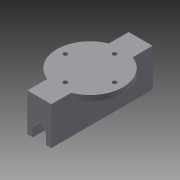
# Autodesk Inventor part: CarFrontAxel
Saved by Autodesk Inventor 2015 (Build 190159000, 159)
## iProperties
Created: 2016-04-06
Part Number: CarFrontAxel
Material: Generic
Document SubType Name: Modeling
Designer: Lee
Density: 1 g/cm^3
Appearance: Default
Author: Lee
Autodesk Inventor part; units mm, degrees
ref_plane "YZ Plane" through (0, 0, 0) normal (1, 0, 0) x (0, 1, 0)
ref_plane "XZ Plane" through (0, 0, 0) normal (0, 1, 0) x (-1, 0, 0)
ref_plane "XY Plane" through (0, 0, 0) normal (0, 0, 1) x (1, 0, 0)
sketch "Sketch1" plane through (0, 0, 0) normal (0, 0, 1) x (1, 0, 0)
  line L0 (0, 0) -> (7.2, 0)
  line L1 (7.2, 0) -> (7.2, 30.48)
  line L2 (7.2, 30.48) -> (0, 30.48)
  line L3 (0, 30.48) -> (0, 0)
  line L4 (5.6, 28.88) -> (5.6, 1.6)
  line L5 (5.6, 1.6) -> (1.6, 1.6)
  line L6 (1.6, 1.6) -> (1.6, 28.88)
  line L7 (1.6, 28.88) -> (5.6, 28.88)
  dimension "d0" = 30.48
  dimension "d1" = 7.2
  dimension "d2" = 1.6
  constraints: 16 end point, 4 parallel, 2 perpendicular, 1 horizontal, 3 other
  measures "d0" distance of L0.end L1.end
  measures "d1" distance of L0.start L0.end
  measures "d2" distance between parallel lines of L1 L4
extrude "Extrusion1" add sketch "Sketch1" along normal blind 11.4
sketch "Sketch2" plane through (0, 0, 0) normal (0, -1, 0) x (1, 0, 0)
  line L0 (5.6, 0) -> (5.6, 11.4) projected
  line L1 (1.6, 0) -> (1.6, 11.4) projected
  line L2 (0, 0) -> (7.2, 0) projected
  line L3 (1.6, 0) -> (1.6, 2.4)
  line L4 (1.6, 0) -> (1.6, 11.4) projected
  line L5 (5.6, 0) -> (5.6, 2.4)
  line L6 (5.6, 0) -> (5.6, 11.4) projected
  line L7 (1.6, 0) -> (5.6, 0)
  arc A0 (5.6, 2.4) -> (1.6, 2.4) centre (3.6, 2.4) ccw
  dimension "d5" = 2.4
  dimension "d6" = 2.4
  constraints: 6 end point, 2 point on circle, 2 point on line, 1 centre point, 1 tangent
  measures "d5" distance of L1.start L3.end
  measures "d6" distance of L0.start L5.end
extrude "Extrusion2" cut sketch "Sketch2" against normal up to surface (30.48 mm away)
sketch "Sketch3" plane through (0, 0, 0) normal (-1, 0, 0) x (0, 0, 1)
  line L0 (0, 30.48) -> (0, 0) projected
  line L1 (0, 0) -> (11.4, 0) projected
  line L2 (11.4, 30.48) -> (11.4, 0) projected
  line L3 (0, 30.48) -> (11.4, 30.48) projected
  line L4 (0, 0) -> (11.4, 0) projected
  line L5 (11.4, 30.48) -> (9.8, 30.48)
  line L6 (9.8, 30.48) -> (9.8, 0)
  line L7 (9.8, 0) -> (11.4, 0)
  line L8 (11.4, 0) -> (11.4, 30.48)
  dimension "d9" = 1.6
  constraints: 8 end point, 2 parallel, 1 horizontal, 1 perpendicular, 1 point on line
  measures "d9" distance of L7.end L6.end
extrude "Extrusion3" add sketch "Sketch3" against normal up to next contours L3 L2 L1 L6
sketch "Sketch4" plane through (0, 0, 11.4) normal (0, 0, 1) x (1, 0, 0)
  line L0 (0, 0) -> (7.2, 0) projected
  line L1 (7.2, 0) -> (7.2, 30.48) projected
  line L2 (7.2, 30.48) -> (0, 30.48) projected
  line L3 (0, 30.48) -> (0, 0) projected
  line L4 (5.6, 0) -> (1.6, 0) projected
  line L5 (3.6, 0) -> (3.6, 30.48)
  line L6 (1.6, 30.48) -> (5.6, 30.48) projected
  line L7 (7.2, 0) -> (0, 30.48)
  line L8 (7.2, 30.48) -> (0, 0) construction
  circle A0 centre (3.6, 7.84) radius 0.65
  circle A1 centre (3.6, 22.64) radius 0.65
  point P0 (3.6, 15.24)
  dimension "d12" = 7.4
  dimension "d13" = 7.4
  dimension "d14" = 1.3
  dimension "d15" = 1.3
  constraints: 6 end point, 3 midpoint, 2 centre point, 2 point on line
  measures "d12" distance of point (3.6, 15.24) A0.centre
  measures "d13" distance of point (3.6, 15.24) A1.centre
  measures "d14" diameter of A0
  measures "d15" diameter of A1
extrude "Extrusion4" cut sketch "Sketch4" against normal up to next contours A0 L5 | L5 A0 | A1 L5 | L5 A1
sketch "Sketch5" plane through (0, 0, 11.4) normal (0, 0, 1) x (1, 0, 0)
  circle A0 centre (3.6, 7.84) radius 0.65 projected
  circle A1 centre (3.6, 22.64) radius 0.65 projected
  line L0 (0, 0) -> (7.2, 0) projected
  line L1 (7.2, 0) -> (7.2, 30.48) projected
  line L2 (7.2, 30.48) -> (0, 30.48) projected
  line L3 (0, 30.48) -> (0, 0) projected
  line L4 (7.2, 0) -> (0, 30.48)
  line L5 (0, 0) -> (7.2, 30.48)
  circle A2 centre (3.6, 15.24) radius 9.935
  dimension "d18" = 19.87
  constraints: 4 end point, 1 centre point, 1 coincident, 1 midpoint
  measures "d18" diameter of A2
extrude "Extrusion5" add sketch "Sketch5" against normal blind 1.6 contours A2 L3 | L3 A2 L4 L5 | L5 L4 A2 | A2 L4 L5 L1 | L1 A2 | L4 A2 L5
sketch "Sketch6" plane through (0, 0, 11.4) normal (0, 0, 1) x (1, 0, 0)
  line L0 (1.6, 28.88) -> (1.6, 1.6) projected
  circle A0 centre (3.6, 22.64) radius 0.65 projected
  circle A1 centre (3.6, 7.84) radius 0.65 projected
  line L1 (0, 5.9802) -> (0, 0) projected
  line L2 (0, 0) -> (7.2, 0) projected
  line L3 (7.2, 0) -> (7.2, 5.9802) projected
  arc A2 (7.2, 5.9802) -> (7.2, 24.4998) centre (3.6, 15.24) ccw projected
  line L4 (7.2, 24.4998) -> (7.2, 30.48) projected
  line L5 (7.2, 30.48) -> (0, 30.48) projected
  line L6 (0, 30.48) -> (0, 24.4998) projected
  arc A3 (0, 24.4998) -> (0, 5.9802) centre (3.6, 15.24) ccw projected
  line L7 (7.2, 0) -> (0, 30.48)
  line L8 (7.2, 30.48) -> (0, 0)
  arc A4 (0, 24.4998) -> (0, 5.9802) centre (3.6, 15.24) ccw projected
  line L9 (-6.335, 15.24) -> (13.535, 15.24) construction
  arc A5 (7.2, 5.9802) -> (7.2, 24.4998) centre (3.6, 15.24) ccw projected
  circle A6 centre (-3.8, 15.24) radius 0.65
  circle A7 centre (11, 15.24) radius 0.65
  dimension "d21" = 7.4
  dimension "d22" = 7.4
  dimension "d23" = 1.3
  dimension "d24" = 1.3
  constraints: 6 end point, 4 point on circle, 2 centre point, 2 point on line
  measures "d21" distance of A2.centre A6.centre
  measures "d22" distance of A2.centre A7.centre
  measures "d23" diameter of A6
  measures "d24" diameter of A7
extrude "Extrusion6" cut sketch "Sketch6" against normal up to next contours A6 | A7
body "Solid1"
